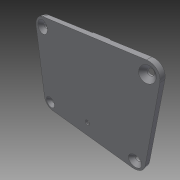
# Autodesk Inventor part: top
Saved by Autodesk Inventor 2014 (Build 180170000, 170)
## iProperties
Created: 2016-03-25
Part Number: top
Material: Generic
Document SubType Name: Modeling
Designer: buben
Density: 1 g/cm^3
Appearance: Default
Author: buben
Autodesk Inventor part; units mm, degrees
ref_plane "YZ Plane" through (0, 0, 0) normal (1, 0, 0) x (0, 1, 0)
ref_plane "XZ Plane" through (0, 0, 0) normal (0, 1, 0) x (-1, 0, 0)
ref_plane "XY Plane" through (0, 0, 0) normal (0, 0, 1) x (1, 0, 0)
sketch "Sketch1" plane through (0, 0, 0) normal (0, 1, 0) x (-1, 0, 0)
  line L0 (0, 0) -> (-66.5, 0)
  line L1 (-66.5, 0) -> (-66.5, -52.5)
  line L2 (-66.5, -52.5) -> (0, -52.5)
  line L3 (0, -52.5) -> (0, 0)
  dimension "d0" = 52.5
  dimension "d1" = 66.5
  constraints: 8 end point, 2 parallel, 1 horizontal, 1 perpendicular
  measures "d0" distance of L2.end L0.start
  measures "d1" distance of L0.start L0.end
extrude "Extrusion1" add sketch "Sketch1" along normal blind 3
sketch "Sketch2" plane through (0, 3, 0) normal (0, 1, 0) x (1, 0, 0)
  line L0 (0, 0) -> (66.5, 0) projected
  line L1 (66.5, 0) -> (66.5, 52.5) projected
  line L2 (33.31, 0) -> (42.31, 0)
  line L3 (42.31, 0) -> (42.31, 3)
  line L4 (42.31, 3) -> (33.31, 3)
  line L5 (33.31, 3) -> (33.31, 0)
  point P0 (37.81, 3)
  dimension "d5" = 9
  dimension "d6" = 3
  dimension "d7" = 28.69
  constraints: 8 end point, 2 parallel, 1 horizontal, 1 midpoint, 1 perpendicular, 1 point on line
  measures "d5" distance of L3.end L4.end
  measures "d6" distance of L4.end L2.start
  measures "d7" distance from line of L1 point (37.81, 3)
extrude "Extrusion2" add sketch "Sketch2" along normal blind 0.4
sketch "Sketch4" plane through (0, 0, 0) normal (0, -1, 0) x (1, 0, 0)
  line L0 (66.5, -52.5) -> (0, -52.5) projected
  line L1 (66.5, 0) -> (66.5, -52.5) projected
  line L2 (61.5, -47.5) -> (5, -47.5) construction
  line L3 (5, -47.5) -> (5, -5) construction
  line L4 (5, -5) -> (61.5, -5) construction
  line L5 (61.5, -5) -> (61.5, -47.5) construction
  point P0 (33.25, -47.5)
  point P1 (33.25, -52.5)
  point P2 (61.5, -26.25)
  point P3 (66.5, -26.25)
  dimension "d12" = 56.5
  dimension "d13" = 42.5
  constraints: 8 end point, 4 coincident, 4 midpoint, 2 parallel, 1 horizontal, 1 horizontal alignment, 1 perpendicular, 1 vertical alignment
  measures "d12" distance of L2.start L2.end
  measures "d13" distance of L4.end L2.start
hole "Hole1" at (61.5, 0, -47.5) at (5, 0, -47.5) at (5, 0, -5) at (61.5, 0, -5) direction (0, 1, 0) diameter 3 end through all countersink diameter 7 countersink angle 90
sketch "Sketch5" plane through (0, 3, 0) normal (0, 1, 0) x (1, 0, 0)
  line L0 (66.5, 52.5) -> (0, 52.5) projected
  line L1 (0, 52.5) -> (0, 0) projected
  line L2 (56.11, 3.39) -> (10.39, 3.39) construction
  line L3 (10.39, 3.39) -> (10.39, 49.11) construction
  line L4 (10.39, 49.11) -> (56.11, 49.11) construction
  line L5 (56.11, 49.11) -> (56.11, 3.39) construction
  point P0 (33.25, 49.11)
  point P1 (33.25, 52.5)
  point P2 (10.39, 26.25)
  point P3 (0, 26.25)
  point P4 (33.25, 44.11)
  dimension "d21" = 45.72
  dimension "d22" = 5
  dimension "d23" = 22.86
  constraints: 8 end point, 4 midpoint, 2 parallel, 2 perpendicular, 1 horizontal, 1 horizontal alignment, 1 vertical alignment
  measures "d21" distance of L2.end L3.end
  measures "d22" distance from line of L4 point (33.25, 44.11)
  measures "d23" distance from line of L3 point (33.25, 44.11)
hole "Hole2" at (33.25, 3, -44.11) direction (0, -1, 0) diameter 3 end through all countersink diameter 8 countersink angle 90
fillet "Fillet1" radius 6 4 edges at (0, 1.5, -52.5) (66.5, 1.5, -52.5) (66.5, 1.5, 0) (0, 1.5, 0)
body "Solid1"
